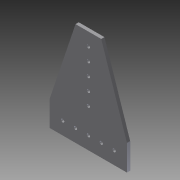
# Autodesk Inventor part: 8 ball frame gusset
Saved by Autodesk Inventor 2012 (Build 160160000, 160)
## iProperties
Created: 2013-12-03
Part Number: 8 ball frame gusset
Material: Default
Document SubType Name: Modeling
Designer: Bryce
Density: 1 g/cm^3
Author: Bryce
Autodesk Inventor part; units mm, degrees
ref_plane "YZ Plane" through (0, 0, 0) normal (1, 0, 0) x (0, 1, 0)
ref_plane "XZ Plane" through (0, 0, 0) normal (0, 1, 0) x (-1, 0, 0)
ref_plane "XY Plane" through (0, 0, 0) normal (0, 0, 1) x (1, 0, 0)
sketch "Sketch1" plane through (0, 0, 0) normal (0, 0, 1) x (1, 0, 0)
  line L0 (0, 0) -> (76.2, 0)
  line L1 (76.2, 0) -> (76.2, 25.4)
  line L2 (76.2, 25.4) -> (50.8, 101.6)
  line L3 (50.8, 101.6) -> (25.4, 101.6)
  line L4 (25.4, 101.6) -> (0, 25.4)
  line L5 (0, 25.4) -> (0, 0)
  line L6 (0, 25.4) -> (76.2, 25.4) construction
  line L7 (25.4, 101.6) -> (25.4, 25.4) construction
  line L8 (50.8, 101.6) -> (50.8, 25.4) construction
  circle A0 centre (12.7, 12.7) radius 1.5875
  circle A1 centre (25.4, 12.7) radius 1.5875
  circle A2 centre (38.1, 12.7) radius 1.5875
  circle A3 centre (50.8, 12.7) radius 1.5875
  circle A4 centre (63.5, 12.7) radius 1.5875
  circle A5 centre (38.1, 88.7759) radius 1.5875
  circle A6 centre (38.1, 76.0759) radius 1.5875
  circle A7 centre (38.1, 63.3759) radius 1.5875
  circle A8 centre (38.1, 50.6759) radius 1.5875
  circle A9 centre (38.1, 37.9759) radius 1.5875
  dimension "d0" = 25.4
  dimension "d1" = 76.2
  dimension "d2" = 101.6
  dimension "d3" = 12.7
  dimension "d4" = 12.7
  dimension "d7" = 12.7
  dimension "d12" = 3.175
  dimension "d13" = 12.8241
  dimension "d14" = 12.7
  dimension "d17" = 12.7
  constraints: 18 end point, 10 centre point, 4 perpendicular, 3 equal length, 2 horizontal, 2 parallel, 2 point on line, 1 equal radius, 1 vertical, 16 other
  measures "d0" distance of L4.end L0.start
  measures "d1" distance of L0.start L0.end
  measures "d2" distance between parallel lines of L0 L3
  measures "d3" distance from line of L0 A0.centre
  measures "d4" distance from line of L5 A0.centre
  measures "d7" distance of A0.centre A1.centre
  measures "d12" diameter of A0
  measures "d13" distance from line of L3 A5.centre
  measures "d14" distance from line of L7 A5.centre
  measures "d17" distance of A5.centre A6.centre
extrude "Extrusion1" add sketch "Sketch1" along normal blind 3.175
equation "\"d4\" = d3"
body "Solid1"
